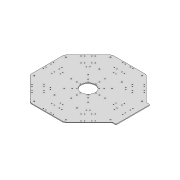
# Autodesk Inventor part: Base
Saved by Autodesk Inventor 2020 (Build 240168000, 168)
## iProperties
Created: 2022-03-01
Part Number: Base
Material: Generic
Document SubType Name: Modeling
Designer: ferrerx
Density: 1 g/cm^3
Appearance: Default
Author: ferrerx
Autodesk Inventor part; units mm, degrees
ref_plane "YZ Plane" through (0, 0, 0) normal (1, 0, 0) x (0, 1, 0)
ref_plane "XZ Plane" through (0, 0, 0) normal (0, 1, 0) x (-1, 0, 0)
ref_plane "XY Plane" through (0, 0, 0) normal (0, 0, 1) x (1, 0, 0)
sketch "Sketch1" plane through (0, 0, 0) normal (0, 1, 0) x (-1, 0, 0)
  circle A0 centre (0, 0) radius 19
  circle A1 centre (0, 0) radius 92.5 construction
  line L0 (115, -37.3658) -> (71.0739, -97.8248) construction
  line L1 (71.0739, -97.8248) -> (0, -120.9182) construction
  line L2 (0, -120.9182) -> (-71.0739, -97.8248) construction
  line L3 (-71.0739, -97.8248) -> (-115, -37.3658) construction
  line L4 (-115, -37.3658) -> (-115, 37.3658) construction
  line L5 (-115, 37.3658) -> (-71.0739, 97.8248) construction
  line L6 (-71.0739, 97.8248) -> (0, 120.9182) construction
  line L7 (0, 120.9182) -> (71.0739, 97.8248) construction
  line L8 (71.0739, 97.8248) -> (115, 37.3658) construction
  line L9 (115, 37.3658) -> (115, -37.3658) construction
  line L10 (0, 0) -> (0, -190.4975) construction
  line L11 (45.5635, -110) -> (-45.5635, -110)
  line L12 (-45.5635, -110) -> (-110, -45.5635)
  line L13 (-110, -45.5635) -> (-110, 45.5635)
  line L14 (-110, 45.5635) -> (-45.5635, 110)
  line L15 (-45.5635, 110) -> (45.5635, 110)
  line L16 (45.5635, 110) -> (110, 45.5635)
  line L17 (110, 45.5635) -> (110, -45.5635)
  line L18 (110, -45.5635) -> (45.5635, -110)
  line L19 (-110, 45.5635) -> (-120, 45.5635)
  line L20 (-120, 45.5635) -> (-120, -45.5635)
  line L21 (-120, -45.5635) -> (-110, -45.5635)
  line L22 (-110, -45.5635) -> (-110, 45.5635)
  dimension "d0" = 38
  dimension "d1" = 185
  dimension "d4" = 230
  dimension "d18" = 220
  dimension "d81" = 10
  constraints: 46 end point, 4 coincident, 4 parallel, 2 centre point, 1 horizontal, 1 perpendicular, 1 vertical, 38 other
  measures "d0" diameter of A0
  measures "d1" diameter of A1
  measures "d4" distance between parallel lines of L4 L9
  measures "d18" distance between parallel lines of L15 L11
  measures "d81" distance of L20.end L21.end
extrude "Extrusion1" add sketch "Sketch1" along normal blind 5
sketch "Sketch2" plane through (0, 5, 0) normal (0, 1, 0) x (1, 0, 0)
  line L0 (0, 0) -> (-95, 0) construction
  line L1 (-106.25, -6.75) -> (-83.75, -6.75) construction
  line L2 (-83.75, -6.75) -> (-83.75, 6.75) construction
  line L3 (-83.75, 6.75) -> (-106.25, 6.75) construction
  line L4 (-106.25, 6.75) -> (-106.25, -6.75) construction
  line L5 (-106.25, -6.75) -> (-83.75, 6.75) construction
  line L6 (-83.75, -6.75) -> (-106.25, 6.75) construction
  circle A0 centre (-106.25, -6.75) radius 1
  circle A1 centre (-106.25, 6.75) radius 1
  circle A2 centre (-83.75, 6.75) radius 1
  circle A3 centre (-83.75, -6.75) radius 1
  line L7 (-115, 37.3658) -> (-115, -37.3658) projected
  line L8 (-110, 45.5635) -> (-110, -45.5635) projected
  dimension "d5" = 22.5
  dimension "d6" = 13.5
  dimension "d7" = 2
  dimension "d8" = 2
  dimension "d9" = 2
  dimension "d10" = 2
  dimension "d19" = 15
  constraints: 14 end point, 4 centre point, 4 coincident, 2 horizontal, 2 midpoint, 2 parallel, 1 perpendicular
  measures "d5" distance of L2.end L3.end
  measures "d6" distance of L3.end L1.start
  measures "d7" diameter of A3
  measures "d8" diameter of A2
  measures "d9" diameter of A1
  measures "d10" diameter of A0
  measures "d19" distance from line of L0.end L8
extrude "Extrusion2" cut sketch "Sketch2" against normal blind 5
pattern_circular "Circular Pattern1" count 8 over 360 about axis through (0, 0, 0) along (0, 1, 0) of "Extrusion2"
fillet "Fillet1" radius 10 6 edges at (-45.5635, 2.5, 110) (45.5635, 2.5, 110) (45.5635, 2.5, -110) (-45.5635, 2.5, -110) (-110, 2.5, -45.5635) (-110, 2.5, 45.5635)
sketch "Sketch3" plane through (0, 5, 0) normal (0, 1, 0) x (1, 0, 0)
  circle A0 centre (-100, -30) radius 1.5 construction
  line L0 (-110, 41.4214) -> (-110, -41.4214) projected
  line L1 (0, 0) -> (-110, 0)
  line L2 (0, 0) -> (-110, 0)
  line L3 (-110, 0) -> (-134, 0) construction
  circle A1 centre (-100, 30) radius 1.5 construction
  arc A2 (-110, -41.4214) -> (-107.0711, -48.4924) centre (-100, -41.4214) ccw projected
  line L4 (0, 0) -> (-100, -41.4214) construction
  line L5 (-100, -41.4214) -> (-109.2354, -45.2564) construction
  circle A3 centre (-102, -42.2498) radius 1.55
  dimension "d22" = 3
  dimension "d23" = 30
  dimension "d24" = 10
  dimension "d30" = 3.1
  dimension "d31" = 102
  constraints: 10 end point, 3 centre point, 1 horizontal, 1 midpoint, 1 point on circle, 1 point on line, 1 symmetric about line, 1 other
  measures "d22" diameter of A0
  measures "d23" vertical distance of L1.start A0.centre
  measures "d24" distance from line of L0 A0.centre
  measures "d30" diameter of A3
  measures "d31" horizontal distance of L1.start A3.centre
extrude "Extrusion3" cut sketch "Sketch3" against normal blind 10
pattern_circular "Circular Pattern2" count 8 over 360 about axis through (0, 0, 0) along (0, 1, 0) of "Extrusion3"
sketch "Sketch4" plane through (0, 5, 0) normal (0, 1, 0) x (1, 0, 0)
  circle A0 centre (-6.75, -83.75) radius 1 projected
  circle A1 centre (6.75, -83.75) radius 1 projected
  line L0 (-6.75, -83.75) -> (6.75, -83.75) construction
  line L1 (0, -83.75) -> (0, -21.25) construction
  circle A2 centre (0, -21.25) radius 1
  point P0 (0, 0)
  dimension "d32" = 62.5
  dimension "d33" = 2
  constraints: 4 end point, 1 centre point, 1 coincident, 1 midpoint, 1 vertical
  measures "d32" distance of L1.start L1.end
  measures "d33" diameter of A2
extrude "Extrusion4" cut sketch "Sketch4" against normal blind 10 contours A2
pattern_circular "Circular Pattern3" count 8 over 360 about axis through (0, 0, 0) along (0, 1, 0) of "Extrusion4"
sketch "Sketch5" plane through (0, 5, 0) normal (0, 1, 0) x (1, 0, 0)
  line L0 (30, -60) -> (-30, -60) construction
  line L1 (-30, -60) -> (-30, 60) construction
  line L2 (-30, 60) -> (30, 60) construction
  line L3 (30, 60) -> (30, -60) construction
  line L4 (30, -60) -> (-30, 60) construction
  line L5 (-30, -60) -> (30, 60) construction
  circle A0 centre (-30, -60) radius 1.5
  circle A1 centre (-30, 60) radius 1.5
  circle A2 centre (30, 60) radius 1.5
  circle A3 centre (30, -60) radius 1.5
  point P0 (0, 0)
  dimension "d39" = 60
  dimension "d40" = 120
  dimension "d41" = 3
  dimension "d42" = 3
  dimension "d43" = 3
  dimension "d44" = 3
  constraints: 12 end point, 4 centre point, 4 coincident, 2 midpoint, 2 parallel, 1 horizontal, 1 perpendicular
  measures "d39" distance of L1.end L2.end
  measures "d40" distance of L2.end L0.start
  measures "d41" diameter of A0
  measures "d42" diameter of A1
  measures "d43" diameter of A2
  measures "d44" diameter of A3
extrude "Extrusion5" cut sketch "Sketch5" against normal blind 10
sketch "Sketch6" plane through (0, 0, 0) normal (0, -1, 0) x (1, 0, 0)
  circle A0 centre (0, 0) radius 172.4819
  constraints: 1 centre point, 1 coincident
extrude "Extrusion6" cut sketch "Sketch6" against normal blind 3
sketch "Sketch7" plane through (0, 5, 0) normal (0, 1, 0) x (1, 0, 0)
  circle A0 centre (-6.75, -106.25) radius 1 construction
  circle A1 centre (6.75, -106.25) radius 1 construction
  line L0 (-6.75, -106.25) -> (6.75, -106.25) construction
  circle A2 centre (-6.75, -83.75) radius 1 construction
  circle A3 centre (6.75, -83.75) radius 1 construction
  line L1 (-6.75, -83.75) -> (6.75, -83.75) construction
  line L2 (0, -106.25) -> (0, -83.75) construction
  line L3 (-13.5, -83.75) -> (13.5, -83.75) construction
  line L4 (13.5, -83.75) -> (13.5, -106.25) construction
  line L5 (13.5, -106.25) -> (-13.5, -106.25) construction
  line L6 (-13.5, -106.25) -> (-13.5, -83.75) construction
  line L7 (-13.5, -83.75) -> (13.5, -106.25) construction
  line L8 (13.5, -83.75) -> (-13.5, -106.25) construction
  circle A4 centre (-13.5, -83.75) radius 1.05
  circle A5 centre (13.5, -83.75) radius 1.05
  circle A6 centre (13.5, -106.25) radius 1.05
  circle A7 centre (-13.5, -106.25) radius 1.05
  point P0 (0, 0)
  point P1 (0, -95)
  dimension "d49" = 22.5
  dimension "d50" = 27
  dimension "d51" = 2.1
  dimension "d52" = 2.1
  dimension "d53" = 2.1
  dimension "d54" = 2.1
  constraints: 18 end point, 5 midpoint, 4 centre point, 4 coincident, 3 horizontal, 2 parallel, 1 perpendicular
  measures "d49" distance of L3.end L4.end
  measures "d50" distance of L3.start L3.end
  measures "d51" diameter of A4
  measures "d52" diameter of A5
  measures "d53" diameter of A6
  measures "d54" diameter of A7
extrude "Extrusion7" cut sketch "Sketch7" against normal blind 3
pattern_circular "Circular Pattern4" count 8 over 360 about axis through (0, 0, 0) along (0, 1, 0) of "Extrusion7"
sketch "Sketch8" plane through (0, 5, 0) normal (0, 1, 0) x (1, 0, 0)
  circle A0 centre (-6.75, -83.75) radius 1 projected
  circle A1 centre (6.75, -83.75) radius 1 projected
  line L0 (-6.75, -83.75) -> (6.75, -83.75) construction
  line L1 (0, -83.75) -> (0, -71.25) construction
  circle A2 centre (-3.25, -71.25) radius 1
  line L2 (-3.25, -71.25) -> (0, -71.25) construction
  circle A3 centre (3.25, -71.25) radius 1
  line L3 (0, -71.25) -> (0, -45.25) construction
  circle A4 centre (0, -45.25) radius 1.25
  circle A5 centre (0, -30.25) radius 1.25
  line L4 (0, -45.25) -> (0, -30.25) construction
  point P0 (0, 0)
  dimension "d60" = 2
  dimension "d61" = 3.25
  dimension "d62" = 12.5
  dimension "d63" = 26
  dimension "d64" = 2.5
  dimension "d65" = 2.5
  dimension "d66" = 15
  constraints: 10 end point, 4 centre point, 2 horizontal, 2 vertical, 1 coincident, 1 midpoint, 1 symmetric about line, 1 other
  measures "d60" diameter of A2
  measures "d61" distance from line of L1 L2.start
  measures "d62" distance between parallel lines of L0 L2
  measures "d63" distance of L1.end L4.start
  measures "d64" diameter of A4
  measures "d65" diameter of A5
  measures "d66" distance of L4.start L4.end
extrude "Extrusion8" cut sketch "Sketch8" against normal blind 10 contours A2 | A3 | A4 | A5
pattern_circular "Circular Pattern5" count 8 over 360 about axis through (0, 0, 0) along (0, 1, 0) of "Extrusion8"
fillet "Fillet2" radius 2 4 edges at (110, 4, -45.5635) (110, 4, 45.5635) (120, 4, 45.5635) (120, 4, -45.5635)
body "Solid1"
